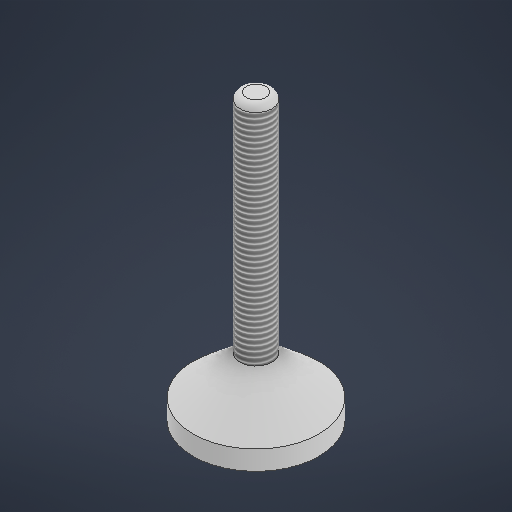
# Autodesk Inventor part: Pied
Saved by Autodesk Inventor 2026.2 (Build 302298010, 298A)
## iProperties
Created: 2026-05-02
Part Number: Pied
Material: Générique
Document SubType Name: Modeling
Designer: romai
Density: 1 g/cm^3
Appearance: Par défaut
Author: romai
Autodesk Inventor part; units mm, degrees
ref_plane "YZ Plane" through (0, 0, 0) normal (1, 0, 0) x (0, 1, 0)
ref_plane "XZ Plane" through (0, 0, 0) normal (0, 1, 0) x (-1, 0, 0)
ref_plane "XY Plane" through (0, 0, 0) normal (0, 0, 1) x (1, 0, 0)
sketch "Esquisse1" plane through (0, 0, 0) normal (0, 0, 1) x (1, 0, 0)
  line L0 (0, 43.5681) -> (0, -28.9477)
  line L1 (0, 0) -> (9.75, 0)
  line L2 (9.75, 0) -> (9.75, 3)
  line L3 (9.75, 3) -> (2.5, 9)
  line L4 (2.5, 9) -> (2.5, 44)
  line L5 (2.5, 44) -> (0, 44)
  line L6 (0, 44) -> (0, 0)
  dimension "d1" = 3
  dimension "d2" = 44
  dimension "d3" = 35
  dimension "d4" = 9.75
  dimension "d5" = 2.5
  constraints: 14 end point, 2 perpendicular, 1 collinear, 1 horizontal, 1 parallel, 1 vertical
  measures "d1" distance of L1.end L2.end
  measures "d2" distance between parallel lines of L1 L5
  measures "d3" distance of L3.end L4.end
  measures "d4" distance of L1.start L1.end
  measures "d5" distance of L4.end L5.end
revolve "Révolution1" add sketch "Esquisse1" angle 360 about axis through (0, 43.5681, 0) along (0, -1, 0)
thread "Filetage1" size "M5x0.8" class "6g" standard "ANSI Metric M Profile" full length
fillet "Congé1" radius 1 1 edges at (-2.5, 44, 0)
